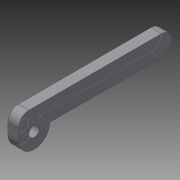
# Autodesk Inventor part: Battery holder
Saved by Autodesk Inventor 2015 (Build 190159000, 159)
## iProperties
Created: 2014-11-13
Part Number: Battery holder
Material: Generic
Document SubType Name: Modeling
Designer: karl
Density: 1 g/cm^3
Appearance: Default
Author: karl
Autodesk Inventor part; units mm, degrees
ref_plane "YZ Plane" through (0, 0, 0) normal (1, 0, 0) x (0, 1, 0)
ref_plane "XZ Plane" through (0, 0, 0) normal (0, 1, 0) x (-1, 0, 0)
ref_plane "XY Plane" through (0, 0, 0) normal (0, 0, 1) x (1, 0, 0)
sketch "Sketch1" plane through (0, 0, 0) normal (1, 0, 0) x (0, 1, 0)
  line L0 (-4.5, 3) -> (4.5, 3)
  line L1 (4.5, 3) -> (4.5, -3)
  line L2 (4.5, -3) -> (-4.5, -3)
  line L3 (-4.5, -3) -> (-4.5, 3)
  line L4 (-4.5, 3) -> (4.5, -3) construction
  line L5 (4.5, 3) -> (-4.5, -3) construction
  circle A0 centre (0, -3) radius 4.5
  point P0 (0, 0)
  dimension "d0" = 9
  dimension "d1" = 6
  dimension "d2" = 9
  constraints: 12 end point, 3 midpoint, 2 parallel, 1 centre point, 1 horizontal, 1 perpendicular
  measures "d0" distance of L1.end L2.end
  measures "d1" distance of L0.end L1.end
  measures "d2" diameter of A0
extrude "Extrusion1" add sketch "Sketch1" along normal blind 3
sketch "Sketch2" plane through (3, 0, 0) normal (1, 0, 0) x (0, 0, -1)
  line L0 (3, 4.5) -> (-3, 4.5)
  line L1 (-3, 4.5) -> (-3, 42.5)
  line L2 (-3, 42.5) -> (3, 42.5)
  line L3 (3, 42.5) -> (3, 4.5)
  point P0 (0, 0)
  dimension "d5" = 6
  dimension "d6" = 38
  constraints: 8 end point, 2 parallel, 1 horizontal, 1 perpendicular
  measures "d5" distance of L1.end L2.end
  measures "d6" distance of L0.end L1.end
extrude "Extrusion2" add sketch "Sketch2" against normal blind 3
sketch "Sketch3" plane through (3, 0, 0) normal (1, 0, 0) x (0, 0, -1)
  arc A0 (3, -4.5) -> (3, 4.5) centre (3, 0) ccw projected
  circle A1 centre (3, 0) radius 1.5
  point P0 (0, 0)
  dimension "d9" = 3
  constraints: 1 centre point, 1 coincident
  measures "d9" diameter of A1
extrude "Extrusion3" cut sketch "Sketch3" against normal blind 3
fillet "Fillet1" radius 3 3 edges at (1.5, -4.5, 3) (1.5, 42.5, 3) (1.5, 42.5, -3)
sketch "Sketch4" plane through (0, 0, 0) normal (-1, 0, 0) x (0, 0, 1)
  circle A0 centre (-3, 38) radius 1.5
  circle A1 centre (-3, 0) radius 1.5 projected
  point P0 (0, 0)
  dimension "d13" = 3
  dimension "d14" = 38
  constraints: 1 centre point, 1 vertical alignment
  measures "d13" diameter of A0
  measures "d14" distance of A1.centre A0.centre
extrude "Extrusion4" cut sketch "Sketch4" against normal blind 3 contours A0
body "Solid1"
